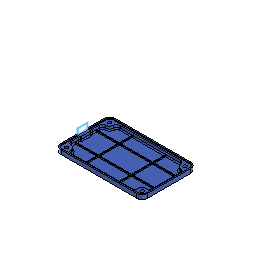
Glasgow_base (Autodesk Fusion 360 design; units mm, degrees)
Autodesk Fusion 360 part; units mm, degrees
note: some values were not read from the file. Chosen so that the rebuilt part matches the saved one: a side. Set by a fixed rule: which sketch regions a step uses.
sketch "Sketch1" plane through (0, 0, 0) normal (0, 0, -1) x (1, 0, 0)
  arc A0 (4, 0) -> (0, -4) centre (4, -4) ccw construction
  line L0 (0, -4) -> (0, -19.9) construction
  line L1 (0, -19.9) -> (0.3, -19.9) construction
  arc A1 (0.7, -20.3) -> (0.3, -19.9) centre (0.3, -20.3) ccw construction
  line L2 (0.7, -20.3) -> (0.7, -28.7) construction
  arc A2 (0.3, -29.1) -> (0.7, -28.7) centre (0.3, -28.7) ccw construction
  line L3 (0.3, -29.1) -> (0, -29.1) construction
  line L4 (0, -29.1) -> (0, -45) construction
  arc A3 (0, -45) -> (4, -49) centre (4, -45) ccw construction
  line L5 (4, -49) -> (76, -49) construction
  arc A4 (76, -49) -> (80, -45) centre (76, -45) ccw construction
  line L6 (80, -45) -> (80, -4) construction
  arc A5 (80, -4) -> (76, 0) centre (76, -4) ccw construction
  line L7 (76, 0) -> (4, 0) construction
  circle A6 centre (52.73, -6.81) radius 0.5 construction
  circle A7 centre (57.81, -42.27) radius 0.5 construction
  circle A8 centre (55.27, -42.27) radius 0.5 construction
  circle A9 centre (52.73, -42.27) radius 0.5 construction
  circle A10 centre (42.57, -42.27) radius 0.5 construction
  circle A11 centre (20.27, -24.5) radius 0.15 construction
  circle A12 centre (20.27, -23.23) radius 0.15 construction
  circle A13 centre (21.54, -24.5) radius 0.15 construction
  circle A14 centre (21.54, -21.96) radius 0.15 construction
  circle A15 centre (21.54, -23.23) radius 0.15 construction
  circle A16 centre (20.27, -21.96) radius 0.15 construction
  circle A17 centre (47.65, -6.81) radius 0.5 construction
  circle A18 centre (42.57, -6.81) radius 0.5 construction
  circle A19 centre (50.19, -6.81) radius 0.5 construction
  circle A20 centre (21.54, -27.04) radius 0.15 construction
  circle A21 centre (20.27, -27.04) radius 0.15 construction
  circle A22 centre (21.54, -25.77) radius 0.15 construction
  circle A23 centre (20.27, -25.77) radius 0.15 construction
  circle A24 centre (23.2666, -41.25) radius 0.15 construction
  circle A25 centre (23.2666, -40.25) radius 0.15 construction
  circle A26 centre (22.2666, -40.25) radius 0.15 construction
  circle A27 centre (22.2666, -41.25) radius 0.15 construction
  circle A28 centre (32.29, -36.75) radius 0.5 construction
  circle A29 centre (29.75, -36.75) radius 0.5 construction
  circle A30 centre (19, -23.23) radius 0.15 construction
  circle A31 centre (19, -24.5) radius 0.15 construction
  circle A32 centre (19, -25.77) radius 0.15 construction
  circle A33 centre (19, -21.96) radius 0.15 construction
  circle A34 centre (19, -27.04) radius 0.15 construction
  circle A35 centre (17.73, -24.5) radius 0.15 construction
  circle A36 centre (17.73, -23.23) radius 0.15 construction
  circle A37 centre (17.73, -21.96) radius 0.15 construction
  circle A38 centre (17.73, -25.77) radius 0.15 construction
  circle A39 centre (17.73, -27.04) radius 0.15 construction
  circle A40 centre (62.89, -42.27) radius 0.5 construction
  circle A41 centre (62.89, -44.81) radius 0.5 construction
  circle A42 centre (60.35, -44.81) radius 0.5 construction
  circle A43 centre (50.19, -44.81) radius 0.5 construction
  circle A44 centre (52.73, -44.81) radius 0.5 construction
  circle A45 centre (55.27, -44.81) radius 0.5 construction
  circle A46 centre (76, -4) radius 1.6 construction
  circle A47 centre (62.89, -4.27) radius 0.5 construction
  circle A48 centre (65.43, -4.27) radius 0.5 construction
  circle A49 centre (60.35, -4.27) radius 0.5 construction
  circle A50 centre (42.57, -4.27) radius 0.5 construction
  circle A51 centre (45.11, -4.27) radius 0.5 construction
  circle A52 centre (47.65, -4.27) radius 0.5 construction
  circle A53 centre (52.73, -4.27) radius 0.5 construction
  circle A54 centre (50.19, -4.27) radius 0.5 construction
  circle A55 centre (55.27, -4.27) radius 0.5 construction
  circle A56 centre (57.81, -4.27) radius 0.5 construction
  circle A57 centre (65.43, -6.81) radius 0.5 construction
  circle A58 centre (62.89, -6.81) radius 0.5 construction
  circle A59 centre (60.35, -6.81) radius 0.5 construction
  circle A60 centre (57.81, -6.81) radius 0.5 construction
  circle A61 centre (55.27, -6.81) radius 0.5 construction
  circle A62 centre (45.11, -6.81) radius 0.5 construction
  circle A63 centre (72.5, -15) radius 1.25 construction
  circle A64 centre (76, -45) radius 1.6 construction
  circle A65 centre (65.43, -42.27) radius 0.5 construction
  circle A66 centre (65.43, -44.81) radius 0.5 construction
  circle A67 centre (60.35, -42.27) radius 0.5 construction
  circle A68 centre (42.57, -44.81) radius 0.5 construction
  circle A69 centre (45.11, -44.81) radius 0.5 construction
  circle A70 centre (47.65, -42.27) radius 0.5 construction
  circle A71 centre (45.11, -42.27) radius 0.5 construction
  circle A72 centre (47.65, -44.81) radius 0.5 construction
  circle A73 centre (50.19, -42.27) radius 0.5 construction
  circle A74 centre (57.81, -44.81) radius 0.5 construction
  circle A75 centre (72.5, -35) radius 1.25 construction
  circle A76 centre (16.46, -21.96) radius 0.15 construction
  circle A77 centre (16.46, -23.23) radius 0.15 construction
  circle A78 centre (16.46, -24.5) radius 0.15 construction
  circle A79 centre (16.46, -25.77) radius 0.15 construction
  circle A80 centre (16.46, -27.04) radius 0.15 construction
  circle A81 centre (4, -4) radius 1.6 construction
  circle A82 centre (4, -45) radius 1.6 construction
  arc A83 (0.6, -20.3) -> (0.3, -20) centre (0.3, -20.3) ccw
  line L8 (-0.1, -20) -> (0.3, -20)
  line L9 (-0.1, -4) -> (-0.1, -20)
  arc A84 (4, 0.1) -> (-0.1, -4) centre (4, -4) ccw
  line L10 (76, 0.1) -> (4, 0.1)
  arc A85 (80.1, -4) -> (76, 0.1) centre (76, -4) ccw
  line L11 (80.1, -45) -> (80.1, -4)
  arc A86 (76, -49.1) -> (80.1, -45) centre (76, -45) ccw
  line L12 (4, -49.1) -> (76, -49.1)
  arc A87 (-0.1, -45) -> (4, -49.1) centre (4, -45) ccw
  line L13 (-0.1, -29) -> (-0.1, -45)
  line L14 (0.3, -29) -> (-0.1, -29)
  arc A88 (0.3, -29) -> (0.6, -28.7) centre (0.3, -28.7) ccw
  line L15 (0.6, -20.3) -> (0.6, -28.7)
  circle A89 centre (4, -4) radius 4.1
  circle A90 centre (76, -4) radius 4.1
  circle A91 centre (76, -45) radius 4.1
  circle A92 centre (4, -45) radius 4.1
  line L16 (-1.3, -21.2) -> (-0.6, -21.2) construction
  line L17 (-1.3, -4) -> (-1.3, -21.2)
  arc A93 (4, 1.3) -> (-1.3, -4) centre (4, -4) ccw
  line L18 (76, 1.3) -> (4, 1.3)
  arc A94 (81.3, -4) -> (76, 1.3) centre (76, -4) ccw
  line L19 (81.3, -45) -> (81.3, -4)
  arc A95 (76, -50.3) -> (81.3, -45) centre (76, -45) ccw
  line L20 (4, -50.3) -> (76, -50.3)
  arc A96 (-1.3, -45) -> (4, -50.3) centre (4, -45) ccw
  line L21 (-1.3, -27.8) -> (-1.3, -45)
  line L22 (-0.6, -27.8) -> (-1.3, -27.8) construction
  line L23 (-0.6, -21.2) -> (-0.6, -27.8) construction
  arc A97 (1.9, -20.3) -> (1.2, -18.9771) centre (0.3, -20.3) ccw
  line L24 (1.2, -4) -> (1.2, -18.9771)
  arc A98 (4, -1.2) -> (1.2, -4) centre (4, -4) ccw
  line L25 (76, -1.2) -> (4, -1.2)
  arc A99 (78.8, -4) -> (76, -1.2) centre (76, -4) ccw
  line L26 (78.8, -45) -> (78.8, -4)
  arc A100 (76, -47.8) -> (78.8, -45) centre (76, -45) ccw
  line L27 (4, -47.8) -> (76, -47.8)
  arc A101 (1.2, -45) -> (4, -47.8) centre (4, -45) ccw
  line L28 (1.2, -30.0229) -> (1.2, -45)
  arc A102 (1.2, -30.0229) -> (1.9, -28.7) centre (0.3, -28.7) ccw
  line L29 (1.9, -20.3) -> (1.9, -28.7)
  line L30 (-1.3, -27.8) -> (-1.3, -21.2)
  dimension "d1" = 0.1
  dimension "d2" = 1.3
  dimension "d3" = 1.2
  constraint concentric A0 A89
  constraint coincident A84.start A89
  constraint tangent L10 A89
  constraint concentric A5 A90
  constraint coincident L10.start A90
  constraint tangent L10 A90
  constraint concentric A4 A91
  constraint coincident A86.start A91
  constraint tangent L12 A91
  constraint concentric A3 A92
  constraint coincident L12.start A92
  constraint tangent L12 A92
  constraint perpendicular L16 L30
extrude "Extrude1" add sketch "Sketch1" along normal blind 3.4 contours A83 L8 L9 L13 L14 A88 L15 A89 A92 A97 L24 L28 A102 L29 | A84 A89 L24 A98 L25 | L10 A89 A90 L25 | A89 L24 A98 L25 | A87 A92 L27 A101 L28 | A85 A90 L25 A99 L26 | L12 A91 A92 L27 | A92 L27 A101 L28 | L11 A90 A91 L26 | A90 L25 A99 L26 | A86 A91 L26 A100 L27 | A91 L26 A100 L27 | L17 A93 L18 A94 L19 A95 L20 A96 L21 L30
sketch "Sketch2" plane through (0, 0, -3.4) normal (0, 0, -1) x (1, 0, 0)
  line L0 (1.2, -18.9771) -> (1.2, -6.995) construction
  arc A0 (1.2, -6.995) -> (6.995, -1.2) centre (4, -4) ccw construction
  line L1 (6.995, -1.2) -> (73.005, -1.2) construction
  arc A1 (73.005, -1.2) -> (78.8, -6.995) centre (76, -4) ccw construction
  line L2 (78.8, -6.995) -> (78.8, -42.005) construction
  arc A2 (78.8, -42.005) -> (73.005, -47.8) centre (76, -45) ccw construction
  line L3 (73.005, -47.8) -> (6.995, -47.8) construction
  arc A3 (6.995, -47.8) -> (1.2, -42.005) centre (4, -45) ccw construction
  line L4 (1.2, -42.005) -> (1.2, -30.0229) construction
  arc A4 (1.2, -30.0229) -> (1.9, -28.7) centre (0.3, -28.7) ccw construction
  line L5 (1.9, -28.7) -> (1.9, -20.3) construction
  arc A5 (1.9, -20.3) -> (1.2, -18.9771) centre (0.3, -20.3) ccw construction
  arc A6 (-1.3, -45) -> (4, -50.3) centre (4, -45) ccw
  line L6 (4, -50.3) -> (76, -50.3)
  arc A7 (76, -50.3) -> (81.3, -45) centre (76, -45) ccw
  line L7 (81.3, -45) -> (81.3, -4)
  arc A8 (81.3, -4) -> (76, 1.3) centre (76, -4) ccw
  line L8 (76, 1.3) -> (4, 1.3)
  arc A9 (4, 1.3) -> (-1.3, -4) centre (4, -4) ccw
  line L9 (-1.3, -4) -> (-1.3, -45)
extrude "Extrude2" add sketch "Sketch2" along normal blind 0.8
chamfer "Chamfer1" distance 1 angle 45 8 edges at (-1.3, 24.5, -4.2) (0.2523, 48.7477, -4.2) (40, 50.3, -4.2) (79.7477, 48.7477, -4.2) (81.3, 24.5, -4.2) (79.7477, 0.2523, -4.2) (40, -1.3, -4.2) (0.2523, 0.2523, -4.2)
fillet "Fillet1" radius 3 10 edges at (6.995, 1.2, -1.7) (1.2, 6.995, -1.7) (1.2, 42.005, -1.7) (6.995, 47.8, -1.7) (1.2, 30.0229, -1.7) (1.2, 18.9771, -1.7) (78.8, 42.005, -1.7) (73.005, 47.8, -1.7) (78.8, 6.995, -1.7) (73.005, 1.2, -1.7)
sketch "Sketch3" plane through (0, 0, 0) normal (0, 0, 1) x (-1, 0, 0)
  circle A0 centre (-4, -45) radius 1.6
  circle A1 centre (-4, -4) radius 1.6
  circle A2 centre (-76, -4) radius 1.6
  circle A3 centre (-76, -45) radius 1.6
extrude "Extrude3" cut sketch "Sketch3" against normal blind 20
sketch "Sketch4" plane through (0, 0, -4.2) normal (0, 0, -1) x (1, 0, 0)
  circle A0 centre (76, -45) radius 1.6
  circle A1 centre (76, -4) radius 1.6
  circle A2 centre (4, -45) radius 1.6
  circle A3 centre (4, -4) radius 1.6
  line L0 (-0.3, -4) -> (-0.3, -45) construction
  arc A4 (-0.3, -45) -> (4, -49.3) centre (4, -45) ccw construction
  line L1 (4, -49.3) -> (76, -49.3) construction
  arc A5 (76, -49.3) -> (80.3, -45) centre (76, -45) ccw construction
  line L2 (80.3, -45) -> (80.3, -4) construction
  arc A6 (80.3, -4) -> (76, 0.3) centre (76, -4) ccw construction
  line L3 (76, 0.3) -> (4, 0.3) construction
  arc A7 (4, 0.3) -> (-0.3, -4) centre (4, -4) ccw construction
  line L4 (74.3834, -42.2) -> (72.7668, -45)
  line L5 (72.7668, -45) -> (74.3834, -47.8)
  line L6 (74.3834, -47.8) -> (77.6166, -47.8)
  line L7 (77.6166, -47.8) -> (79.2332, -45)
  line L8 (79.2332, -45) -> (77.6166, -42.2)
  line L9 (77.6166, -42.2) -> (74.3834, -42.2)
  point P0 (76, -45)
  dimension "d12" = 2.8
  constraint coincident P0 A0.centre
  measures "d12" distance of P0 L9
extrude "Extrude4" cut sketch "Sketch4" against normal blind 2 contours L4 L5 L6 L7 L8 L9
sketch "Sketch7" plane through (0, 0, -2.2) normal (0, 0, -1) x (1, 0, 0)
  line L0 (74.4, -47.7585) -> (77.6, -47.7585)
  line L1 (77.6, -47.7585) -> (77.6, -42.2512)
  line L2 (77.6, -42.2512) -> (74.4, -42.2512)
  line L3 (74.4, -42.2512) -> (74.4, -47.7585)
  line L4 (72.7668, -45) -> (74.3834, -42.2)
  line L5 (74.3834, -42.2) -> (77.6166, -42.2)
  line L6 (77.6166, -42.2) -> (79.2332, -45)
  line L7 (79.2332, -45) -> (77.6166, -47.8)
  line L8 (77.6166, -47.8) -> (74.3834, -47.8)
  line L9 (74.3834, -47.8) -> (72.7668, -45)
  circle A0 centre (76, -4) radius 1.6
  circle A1 centre (4, -45) radius 1.6
  circle A2 centre (4, -4) radius 1.6
  line L10 (-0.3, -4) -> (-0.3, -45)
  arc A3 (-0.3, -45) -> (4, -49.3) centre (4, -45) ccw
  line L11 (4, -49.3) -> (76, -49.3)
  arc A4 (76, -49.3) -> (80.3, -45) centre (76, -45) ccw
  line L12 (80.3, -45) -> (80.3, -4)
  arc A5 (80.3, -4) -> (76, 0.3) centre (76, -4) ccw
  line L13 (76, 0.3) -> (4, 0.3)
  arc A6 (4, 0.3) -> (-0.3, -4) centre (4, -4) ccw
  point P0 (74.4, -45)
  point P1 (77.6, -45)
  constraint horizontal L0
  constraint vertical L1
  constraint horizontal L2
  constraint vertical L3
  constraint coincident L3 P0
  constraint coincident L1 P1
extrude "Extrude7" cut sketch "Sketch7" against normal blind 0.2 contours L0 L1 L2 L3
pattern_linear "R-Pattern1" count 2 spacing 72 along (-1, 0, 0) count 2 spacing 41 along (0, -1, 0) of "Extrude4", "Extrude7"
sketch "Sketch5" plane through (0, 0, 0) normal (0, 0, 1) x (-1, 0, 0)
  circle A0 centre (-76, -45) radius 1.6
  circle A1 centre (-76, -4) radius 1.6
  circle A2 centre (-4, -45) radius 1.6
  circle A3 centre (-4, -4) radius 1.6
  arc A4 (-1.6565, -19.4516) -> (-1.2, -17.8607) centre (-4.2, -17.8607) ccw construction
  arc A5 (-1.6565, -19.4516) -> (-1.9, -20.3) centre (-0.3, -20.3) ccw construction
  line L0 (-1.9, -20.3) -> (-1.9, -28.7) construction
  arc A6 (-1.9, -28.7) -> (-1.6565, -29.5484) centre (-0.3, -28.7) ccw construction
  arc A7 (-1.2, -31.1393) -> (-1.6565, -29.5484) centre (-4.2, -31.1393) ccw construction
  line L1 (-1.2, -31.1393) -> (-1.2, -37.9028) construction
  arc A8 (-4.1155, -40.9016) -> (-1.2, -37.9028) centre (-4.2, -37.9028) ccw construction
  arc A9 (-4.1155, -40.9016) -> (-8.0984, -44.8845) centre (-4, -45) ccw construction
  arc A10 (-11.0972, -47.8) -> (-8.0984, -44.8845) centre (-11.0972, -44.8) ccw construction
  line L2 (-11.0972, -47.8) -> (-68.9028, -47.8) construction
  arc A11 (-71.9016, -44.8845) -> (-68.9028, -47.8) centre (-68.9028, -44.8) ccw construction
  arc A12 (-71.9016, -44.8845) -> (-75.8845, -40.9016) centre (-76, -45) ccw construction
  arc A13 (-78.8, -37.9028) -> (-75.8845, -40.9016) centre (-75.8, -37.9028) ccw construction
  line L3 (-78.8, -37.9028) -> (-78.8, -11.0972) construction
  arc A14 (-75.8845, -8.0984) -> (-78.8, -11.0972) centre (-75.8, -11.0972) ccw construction
  arc A15 (-75.8845, -8.0984) -> (-71.9016, -4.1155) centre (-76, -4) ccw construction
  arc A16 (-68.9028, -1.2) -> (-71.9016, -4.1155) centre (-68.9028, -4.2) ccw construction
  line L4 (-68.9028, -1.2) -> (-11.0972, -1.2) construction
  arc A17 (-8.0984, -4.1155) -> (-11.0972, -1.2) centre (-11.0972, -4.2) ccw construction
  arc A18 (-8.0984, -4.1155) -> (-4.1155, -8.0984) centre (-4, -4) ccw construction
  arc A19 (-1.2, -11.0972) -> (-4.1155, -8.0984) centre (-4.2, -11.0972) ccw construction
  line L5 (-1.2, -11.0972) -> (-1.2, -17.8607) construction
  arc A20 (-4, -50.3) -> (1.3, -45) centre (-4, -45) ccw
  line L6 (1.3, -45) -> (1.3, -4)
  arc A21 (1.3, -4) -> (-4, 1.3) centre (-4, -4) ccw
  line L7 (-4, 1.3) -> (-76, 1.3)
  arc A22 (-76, 1.3) -> (-81.3, -4) centre (-76, -4) ccw
  line L8 (-81.3, -4) -> (-81.3, -45)
  arc A23 (-81.3, -45) -> (-76, -50.3) centre (-76, -45) ccw
  line L9 (-76, -50.3) -> (-4, -50.3)
  line L10 (-4, 0.1) -> (-76, 0.1)
  arc A24 (-76, 0.1) -> (-80.1, -4) centre (-76, -4) ccw
  line L11 (-80.1, -4) -> (-80.1, -45)
  arc A25 (-80.1, -45) -> (-76, -49.1) centre (-76, -45) ccw
  line L12 (-76, -49.1) -> (-4, -49.1)
  arc A26 (-4, -49.1) -> (0.1, -45) centre (-4, -45) ccw
  line L13 (0.1, -45) -> (0.1, -4)
  arc A27 (0.1, -4) -> (-4, 0.1) centre (-4, -4) ccw
  dimension "d19" = 1.2
extrude "Extrude5" add sketch "Sketch5" along normal blind 0.8 contours A20 L6 A21 L7 A22 L8 A23 L9
sketch "sketch 4018" plane through (-1.3, 0, 0) normal (-1, 0, 0) x (0, -1, 0)
  line L0 (-19.8373, 1.6) -> (-19.8373, 5.1077)
  line L1 (-19.8373, 5.1077) -> (-29.1, 5.1077)
  line L2 (-29.1, 5.1077) -> (-29.1, 0)
  line L3 (-29.1, 0) -> (-19.8373, 0)
  line L4 (-19.8373, 0) -> (-19.8373, 1.6)
extrude "Extrude6" cut sketch "sketch 4018" against normal blind 13
chamfer "Chamfer2" distance 0.8 angle 45 2 edges at (-1.3, 29.1, 0.4) (-1.3, 19.8373, 0.4)
chamfer "Chamfer3" distance 0.8 angle 45 1 edges at (-1.3, 24.4687, 0)
sketch "Sketch8" plane through (0, 0, -3.4) normal (0, 0, 1) x (-1, 0, 0)
  line L0 (-1.2, -17.8607) -> (-1.2, -11.0972)
  line L1 (-78.8, -11.0972) -> (-78.8, -37.9028)
  line L2 (-1.2, -14.479) -> (-78.8, -14.479)
  line L3 (-1.2, -37.9028) -> (-1.2, -31.1393)
  line L4 (-1.2, -34.521) -> (-78.8, -34.521)
  line L5 (-68.9028, -47.8) -> (-11.0972, -47.8)
  line L6 (-11.0972, -1.2) -> (-68.9028, -1.2)
  line L7 (-22.8527, -47.8) -> (-22.8527, -1.2)
  line L8 (-55.3739, -1.2) -> (-55.3739, -47.8)
  constraint midpoint L0 L2.start
  constraint coincident L1 L2.end
  constraint perpendicular L1 L2
  constraint midpoint L3 L4.start
  constraint coincident L1 L4.end
  constraint perpendicular L1 L4
  constraint coincident L5 L7.start
  constraint coincident L6 L7.end
  constraint perpendicular L4 L7
  constraint coincident L6 L8.start
  constraint coincident L5 L8.end
  constraint perpendicular L5 L8
fillet "Fillet2" radius 1 22 edges at (6.8991, 42.1009, -3.4) (2.049, 39.994, -3.4) (1.2, 34.521, -3.4) (1.3164, 30.3117, -3.4) (1.8379, 29.1413, -3.4) (1.9, 24.5, -3.4) (1.8379, 19.8587, -3.4) (1.3164, 18.6883, -3.4) (1.2, 14.479, -3.4) (2.049, 9.006, -3.4) (6.8991, 6.8991, -3.4) (9.006, 2.049, -3.4) (40, 1.2, -3.4) (70.994, 2.049, -3.4) (73.1009, 6.8991, -3.4) (77.951, 9.006, -3.4) (78.8, 24.5, -3.4) (77.951, 39.994, -3.4) (73.1009, 42.1009, -3.4) (70.994, 46.951, -3.4) (40, 47.8, -3.4) (9.006, 46.951, -3.4)
rib "Web1" add thickness 0.8 on left direction (0, 0, 1) depth 1 extending the curves path "Sketch8" along L7 L2 L4 L8
equation "d2 = 1.2 mm + 0.1 mm"
equation "d12 = ( 3 * 0.9 ) * 1 mm + 0.1 mm"
